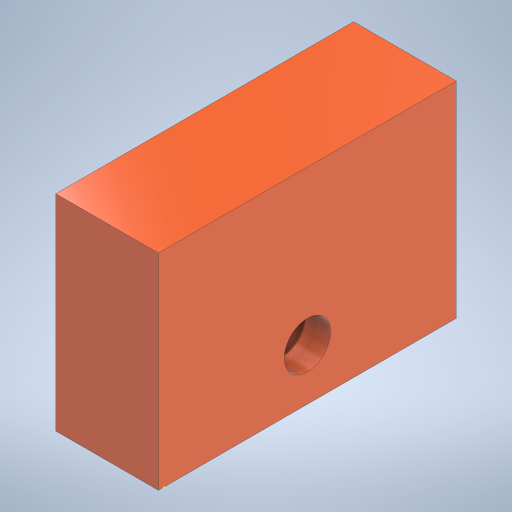
# Autodesk Inventor part: Kolv
Saved by Autodesk Inventor 2024 (Build 280153020, 153B)
## iProperties
Created: 2023-09-13
Part Number: Kolv
Material: Generic
Document SubType Name: Modeling
Designer: 23also
Density: 1 g/cm^3
Appearance: Default
Author: 23also
Autodesk Inventor part; units mm, degrees
ref_plane "YZ Plane" through (0, 0, 0) normal (1, 0, 0) x (0, 1, 0)
ref_plane "XZ Plane" through (0, 0, 0) normal (0, 1, 0) x (-1, 0, 0)
ref_plane "XY Plane" through (0, 0, 0) normal (0, 0, 1) x (1, 0, 0)
sketch "Sketch1" plane through (0, 0, 0) normal (0, 1, 0) x (-1, 0, 0)
  line L0 (0, 0) -> (10, 0)
  line L1 (10, 0) -> (10, -28)
  line L2 (10, -28) -> (0, -28)
  line L3 (0, -28) -> (0, 0)
  constraints: 8 end point, 2 parallel, 1 horizontal, 1 perpendicular
extrude "Extrusion1" add sketch "Sketch1" along normal blind 20
sketch "Sketch6" plane through (0, 0, 0) normal (1, 0, 0) x (0, 0, -1)
  point P0 (0, 0)
sketch "Sketch7" plane through (0, 0, 0) normal (1, 0, 0) x (0, 0, -1)
  circle A0 centre (14, 5) radius 2.25
  point P0 (0, 0)
  dimension "d14" = 4.5
  constraints: 1 centre point
  measures "d14" diameter of A0
extrude "Extrusion6" cut sketch "Sketch7" against normal blind 2.5
sketch "Sketch8" plane through (0, 0, 0) normal (1, 0, 0) x (0, 0, -1)
  line L0 (0, 0) -> (0, 20) projected
  line L1 (0, 0) -> (-0.5, 0)
  line L2 (-0.5, 0) -> (-0.5, 20)
  line L3 (-0.5, 20) -> (0, 20)
  line L4 (0, 20) -> (0, 0)
  line L5 (28, 0) -> (28.5, 0)
  line L6 (28.5, 0) -> (28.5, 20)
  line L7 (28.5, 20) -> (28, 20)
  line L8 (28, 20) -> (28, 0)
  dimension "d17" = 0.5
  dimension "d18" = 0.5
  constraints: 16 end point, 4 parallel, 2 horizontal, 2 perpendicular, 2 point on line
  measures "d17" distance of L2.end L3.end
  measures "d18" distance of L7.end L6.end
extrude "Extrusion7" add sketch "Sketch8" against normal blind 10
body "Solid1"
